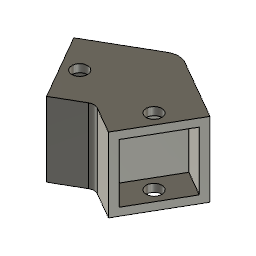
joint (Autodesk Fusion 360 design; units mm, degrees)
Autodesk Fusion 360 part; units mm, degrees
sketch "Sketch1" plane through (0, 0, 0) normal (0, 0, 1) x (1, 0, 0)
  line L0 (0, 0) -> (0, 25.035) construction
  line L1 (0, 25.035) -> (12.9904, 17.535) construction
  circle A0 centre (12.9904, 17.535) radius 2.75
  line L2 (12.9904, 17.535) -> (17.0367, 24.5434) construction
  line L3 (8.6603, 20.035) -> (13.6603, 28.6952)
  line L4 (13.6603, 28.6952) -> (17.9904, 26.1952)
  line L5 (12.9904, 17.535) -> (15.372, 16.16) construction
  line L6 (17.3205, 15.035) -> (22.3205, 23.6952)
  line L7 (22.3205, 23.6952) -> (17.9904, 26.1952)
  line L8 (8.6603, 20.035) -> (3.6603, 11.3747)
  line L9 (3.6603, 11.3747) -> (7.9904, 8.8747)
  line L10 (17.3205, 15.035) -> (12.3205, 6.3747)
  line L11 (12.3205, 6.3747) -> (7.9904, 8.8747)
  line L12 (12.3205, 6.3747) -> (10.8205, 3.7766)
  line L13 (10.8205, 3.7766) -> (0, 10.0239)
  line L14 (0, 25.035) -> (0, 55.0088) construction
  line L15 (22.3205, 23.6952) -> (23.8205, 26.2933)
  line L16 (23.8205, 26.2933) -> (0, 40.0219)
  line L17 (-23.8205, 26.2933) -> (0, 40.0219)
  line L18 (-22.3205, 23.6952) -> (-23.8205, 26.2933)
  line L19 (-22.3205, 23.6952) -> (-17.9904, 26.1952)
  line L20 (-13.6603, 28.6952) -> (-17.9904, 26.1952)
  line L21 (-8.6603, 20.035) -> (-13.6603, 28.6952)
  line L22 (-8.6603, 20.035) -> (-3.6603, 11.3747)
  line L23 (-3.6603, 11.3747) -> (-7.9904, 8.8747)
  line L24 (-12.3205, 6.3747) -> (-7.9904, 8.8747)
  line L25 (-17.3205, 15.035) -> (-12.3205, 6.3747)
  line L26 (-17.3205, 15.035) -> (-22.3205, 23.6952)
  circle A1 centre (-12.9904, 17.535) radius 2.75
  line L27 (-12.3205, 6.3747) -> (-10.8205, 3.7766)
  line L28 (-10.8205, 3.7766) -> (0, 10.0239)
  dimension "d1" = 60
  dimension "d2" = 5.5
  dimension "d3" = 5
  dimension "d4" = 10
  dimension "d5" = 15
  dimension "d7" = 3
  dimension "d8" = 3
  constraint coincident L0.start origin
  constraint vertical L0
  constraint coincident L1.end A0.centre
  constraint perpendicular L1 L2
  constraint perpendicular L1 L3
  constraint coincident L1 L3.start
  constraint coincident L2 L4.end
  constraint perpendicular L2 L4
  constraint coincident A0 L5.end
  constraint perpendicular L2 L5
  constraint symmetric L2 L3.start L6.start
  constraint symmetric L2 L3.end L6.end
  constraint symmetric L2 L4.end L7.end
  constraint symmetric L3.start L5 L8.start
  constraint symmetric L3.end L5 L8.end
  constraint symmetric L4.end L5 L9.end
  constraint symmetric L5 L6.start L10.start
  constraint symmetric L5 L6.end L10.end
  constraint symmetric L5 L4.end L9.end
  constraint perpendicular L11 L12
  constraint coincident L0 L13.end
  constraint parallel L0 L14
  constraint perpendicular L7 L15
  constraint midpoint L14 L16.end
  constraint symmetric L0 A0 A1
  constraint symmetric L0 L3.start L21.start
  constraint symmetric L0 L3.end L20.start
  constraint symmetric L0 L4.end L19.end
  constraint symmetric L0 L6.start L25.start
  constraint symmetric L0 L6.end L18.start
  constraint symmetric L0 L8.end L22.end
  constraint symmetric L0 L9.end L23.end
  constraint symmetric L0 L10.end L24.start
  constraint symmetric L0 L12.end L27.end
  constraint symmetric L0 L13.end L28.end
  constraint symmetric L0 L15.end L17.start
  constraint symmetric L0 L16.end L17.end
  measures "d1" angle of L0 L1
  measures "d2" diameter of A0
  measures "d3" distance of L1.end L3
  measures "d4" distance of L3.start L3.end
  measures "d5" distance of L0.end L1.end
  measures "d7" distance of L10.end L12.end
  measures "d8" distance of L6.end L15.end
extrude "Extrude1" add sketch "Sketch1" along normal blind 26
sketch "Sketch2" plane through (-6.48, -3.7413, 0) normal (-0.866025, -0.5, 0) x (0.5, -0.866025, 0)
  line L0 (-34.6809, 0) -> (-8.6809, 0)
  line L1 (-8.6809, 0) -> (-8.6809, 26)
  line L2 (-8.6809, 26) -> (-34.6809, 26)
  line L3 (-34.6809, 26) -> (-34.6809, 0)
  line L4 (-34.6809, 26) -> (-8.6809, 0) construction
  line L5 (-31.9309, 23.25) -> (-11.4309, 23.25)
  line L6 (-11.4309, 23.25) -> (-11.4309, 2.75)
  line L7 (-11.4309, 2.75) -> (-31.9309, 2.75)
  line L8 (-31.9309, 2.75) -> (-31.9309, 23.25)
  line L9 (-31.9309, 23.25) -> (-11.4309, 2.75) construction
  line L10 (-11.4309, 23.25) -> (-31.9309, 2.75) construction
  point P0 (-21.6809, 13)
  dimension "d11" = 20.5
  dimension "d12" = 20.5
  constraint coincident L2.end L3.start
  constraint coincident L0.end L1.start
  constraint horizontal L5
  constraint perpendicular L5 L6
  constraint parallel L5 L7
  constraint parallel L6 L8
  constraint coincident L9 P0
  constraint coincident L10 P0
  constraint midpoint L4 P0
  measures "d11" distance of L6.end L7.end
  measures "d12" distance of L5.end L6.end
sketch "Sketch3" plane through (6.48, -3.7413, 0) normal (0.866025, -0.5, 0) x (0.5, 0.866025, 0)
  line L0 (8.6809, 0) -> (34.6809, 0)
  line L1 (34.6809, 0) -> (34.6809, 26)
  line L2 (34.6809, 26) -> (8.6809, 26)
  line L3 (8.6809, 26) -> (8.6809, 0)
  line L4 (8.6809, 26) -> (34.6809, 0) construction
  line L5 (31.9309, 23.25) -> (11.4309, 23.25)
  line L6 (11.4309, 23.25) -> (11.4309, 2.75)
  line L7 (11.4309, 2.75) -> (31.9309, 2.75)
  line L8 (31.9309, 2.75) -> (31.9309, 23.25)
  line L9 (31.9309, 23.25) -> (11.4309, 2.75) construction
  line L10 (11.4309, 23.25) -> (31.9309, 2.75) construction
  point P0 (21.6809, 13)
  dimension "d13" = 20.5
  dimension "d14" = 20.5
  constraint coincident L2.end L3.start
  constraint coincident L0.end L1.start
  constraint horizontal L5
  constraint perpendicular L5 L6
  constraint parallel L5 L7
  constraint parallel L6 L8
  constraint coincident L9 P0
  constraint coincident L10 P0
  constraint midpoint L4 P0
  measures "d13" distance of L6.end L7.end
  measures "d14" distance of L5.end L6.end
extrude "Extrude2" cut sketch "Sketch2" against normal blind 10 contours L5 L6 L7 L8
extrude "Extrude3" cut sketch "Sketch3" against normal blind 10 contours L5 L6 L7 L8
fillet "Fillet1" radius 3 1 edges at (0, 10.0239, 13)
fillet "Fillet2" radius 6 1 edges at (0, 40.0219, 13)
equation "d2 = screw"
equation "d5 = dist"
equation "d11 = slot"
equation "d12 = slot"
equation "d13 = slot"
equation "d14 = slot"
equation "dist = 15 mm"
equation "slot = 20.5 mm"
equation "screw = 5.5 mm"
